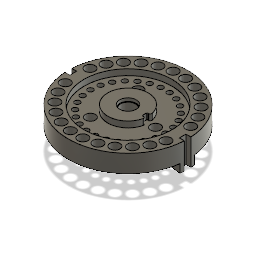
Reverse Roll v5 (Autodesk Fusion 360 design; units mm, degrees)
Autodesk Fusion 360 part; units mm, degrees
sketch "View A" plane through (0, 0, 0) normal (0, 1, 0) x (1, 0, 0)
  circle A0 centre (0, 0) radius 26.45
  circle A1 centre (0, 0) radius 16.6 construction
  circle A2 centre (0, 0) radius 22.6 construction
  circle A3 centre (0, 0) radius 31.25 construction
  circle A4 centre (16.6, 0) radius 3
  circle A5 centre (-8.3, 14.376) radius 3
  circle A6 centre (-8.3, -14.376) radius 3
  circle A7 centre (0, 0) radius 5
  circle A8 centre (0, 0) radius 4.5
  line L0 (10.5, 1.5) -> (10.9174, 1.5)
  line L1 (10.9174, -1.5) -> (10.5, -1.5)
  line L2 (10, -1) -> (10, 1)
  arc A9 (10.5, 1.5) -> (10, 1) centre (10.5, 1) ccw
  arc A10 (10, -1) -> (10.5, -1.5) centre (10.5, -1) ccw
  arc A11 (10.9174, 1.5) -> (11.8922, 2.7232) centre (10.9174, 2.5) ccw
  arc A12 (11.8922, -2.7232) -> (10.9174, -1.5) centre (10.9174, -2.5) ccw
  circle A13 centre (-22.5979, 0) radius 1.6
  circle A14 centre (-22.5979, 0) radius 2
  circle A15 centre (-21.9412, -5.408) radius 2
  circle A16 centre (-21.9412, -5.408) radius 1.6
  circle A17 centre (-20.0094, -10.5017) radius 2
  circle A18 centre (-20.0094, -10.5017) radius 1.6
  circle A19 centre (-16.9148, -14.9851) radius 2
  circle A20 centre (-16.9148, -14.9851) radius 1.6
  circle A21 centre (-12.8371, -18.5977) radius 2
  circle A22 centre (-12.8371, -18.5977) radius 1.6
  circle A23 centre (-8.0133, -21.1294) radius 2
  circle A24 centre (-8.0133, -21.1294) radius 1.6
  circle A25 centre (-2.7239, -22.4331) radius 2
  circle A26 centre (-2.7239, -22.4331) radius 1.6
  circle A27 centre (2.7239, -22.4331) radius 2
  circle A28 centre (2.7239, -22.4331) radius 1.6
  circle A29 centre (8.0133, -21.1294) radius 2
  circle A30 centre (8.0133, -21.1294) radius 1.6
  circle A31 centre (12.837, -18.5977) radius 2
  circle A32 centre (12.837, -18.5977) radius 1.6
  circle A33 centre (16.9147, -14.9852) radius 2
  circle A34 centre (16.9147, -14.9852) radius 1.6
  circle A35 centre (20.0094, -10.5018) radius 2
  circle A36 centre (20.0094, -10.5018) radius 1.6
  circle A37 centre (21.9412, -5.408) radius 2
  circle A38 centre (21.9412, -5.408) radius 1.6
  circle A39 centre (22.5979, 0) radius 2
  circle A40 centre (22.5979, 0) radius 1.6
  circle A41 centre (21.9412, 5.408) radius 2
  circle A42 centre (21.9412, 5.408) radius 1.6
  circle A43 centre (20.0094, 10.5017) radius 2
  circle A44 centre (20.0094, 10.5017) radius 1.6
  circle A45 centre (16.9148, 14.9851) radius 2
  circle A46 centre (16.9148, 14.9851) radius 1.6
  circle A47 centre (12.8371, 18.5977) radius 2
  circle A48 centre (12.8371, 18.5977) radius 1.6
  circle A49 centre (8.0133, 21.1294) radius 2
  circle A50 centre (8.0133, 21.1294) radius 1.6
  circle A51 centre (2.7239, 22.4331) radius 2
  circle A52 centre (2.7239, 22.4331) radius 1.6
  circle A53 centre (-2.7239, 22.4331) radius 2
  circle A54 centre (-2.7239, 22.4331) radius 1.6
  circle A55 centre (-8.0133, 21.1294) radius 2
  circle A56 centre (-8.0133, 21.1294) radius 1.6
  circle A57 centre (-12.837, 18.5977) radius 2
  circle A58 centre (-12.837, 18.5977) radius 1.6
  circle A59 centre (-16.9147, 14.9852) radius 2
  circle A60 centre (-16.9147, 14.9852) radius 1.6
  circle A61 centre (-20.0094, 10.5018) radius 2
  circle A62 centre (-20.0094, 10.5018) radius 1.6
  circle A63 centre (-21.9412, 5.408) radius 2
  circle A64 centre (-21.9412, 5.408) radius 1.6
  circle A65 centre (-31.25, -0.0368) radius 3 construction
  circle A66 centre (-30.3331, -7.5143) radius 3
  circle A67 centre (-27.6534, -14.5552) radius 3
  circle A68 centre (-23.3665, -20.7501) radius 3
  circle A69 centre (-17.7217, -25.7391) radius 3
  circle A70 centre (-11.047, -29.2323) radius 3
  circle A71 centre (-3.7302, -31.0266) radius 3
  circle A72 centre (3.8033, -31.0177) radius 3
  circle A73 centre (11.1158, -29.2062) radius 3
  circle A74 centre (17.7823, -25.6973) radius 3
  circle A75 centre (23.4153, -20.695) radius 3
  circle A76 centre (27.6876, -14.49) radius 3
  circle A77 centre (30.3507, -7.4429) radius 3
  circle A78 centre (31.25, 0.0368) radius 3 construction
  circle A79 centre (30.3331, 7.5143) radius 3
  circle A80 centre (27.6534, 14.5552) radius 3
  circle A81 centre (23.3665, 20.7501) radius 3
  circle A82 centre (17.7217, 25.7391) radius 3
  circle A83 centre (11.047, 29.2323) radius 3
  circle A84 centre (3.7302, 31.0266) radius 3
  circle A85 centre (-3.8033, 31.0177) radius 3
  circle A86 centre (-11.1158, 29.2062) radius 3
  circle A87 centre (-17.7823, 25.6973) radius 3
  circle A88 centre (-23.4153, 20.695) radius 3
  circle A89 centre (-27.6876, 14.49) radius 3
  circle A90 centre (-30.3507, 7.4429) radius 3
  line L3 (-35.9464, 1.9631) -> (-32.9464, 1.9631)
  line L4 (-32.9464, 1.9631) -> (-32.9464, -2.0369)
  line L5 (-32.9464, -2.0369) -> (-35.9423, -2.0369)
  line L6 (35.9464, -1.9631) -> (32.9464, -1.9631)
  line L7 (32.9464, -1.9631) -> (32.9464, 2.0369)
  line L8 (32.9464, 2.0369) -> (35.9423, 2.0369)
  arc A91 (-35.9423, -2.0369) -> (35.9464, -1.9631) centre (0, 0) ccw
  arc A92 (35.9423, 2.0369) -> (-35.9464, 1.9631) centre (0, 0) ccw
  circle A93 centre (0, 0) radius 8.5 construction
  arc A94 (0, 8.5) -> (-4.25, 7.3612) centre (0, 0) ccw
  line L9 (0, 0) -> (0, 8.5) construction
  line L10 (0, 0) -> (-4.25, 7.3612) construction
  circle A95 centre (-4.25, 7.3612) radius 3
  circle A96 centre (-4.25, -7.3612) radius 3
  circle A97 centre (8.5, 0) radius 3
  circle A98 centre (0, 0) radius 12.2
  dimension "d1" = 24.4
  dimension "d2" = 52.9
  dimension "d7" = 6
  dimension "d9" = 360
  dimension "d16" = 0.5
  dimension "d18" = 1
  dimension "d19" = 1
  dimension "d21" = 0.5
  dimension "d25" = 360
  dimension "d26" = 6
  dimension "d28" = 360
  dimension "d30" = 4
  dimension "d32" = 4
  dimension "d37" = 17
  dimension "d38" = 30
  dimension "d39" = 6
  dimension "d41" = 360
  dimension "d126" = 3
  dimension "d127" = 3
  measures "d1" diameter of A98
  measures "d2" diameter of A0
  measures "d7" diameter of A4
  measures "d16" radius of A9
  measures "d18" radius of A11
  measures "d19" radius of A12
  measures "d21" radius of A10
  measures "d26" diameter of A65
  measures "d37" diameter of A93
  measures "d38" angle of L9 L10
  measures "d39" diameter of A95
sketch "View B" plane through (0, 0, 0) normal (0, 1, 0) x (1, 0, 0)
  circle A0 centre (0, 0) radius 12.5
  circle A1 centre (0, 0) radius 17 construction
  circle A2 centre (-15.9748, 5.8143) radius 2
  circle A3 centre (13.0228, 10.9274) radius 2
  circle A4 centre (2.952, -16.7417) radius 2
  arc A5 (-35.9423, -2.0369) -> (35.9464, -1.9631) centre (0, 0) ccw
  line L0 (35.7317, -4.3873) -> (26.7445, -3.2838)
  line L1 (26.175, -3.8044) -> (20.7581, -3.0171)
  line L2 (24.9681, -8.729) -> (19.801, -6.9225)
  line L3 (26.7445, 3.2838) -> (35.7317, 4.3873)
  line L4 (25.3133, -2.4374) -> (14.8977, -1.4345)
  line L5 (25.3133, 2.4374) -> (14.8977, 1.4345)
  arc A6 (26.4075, -1.4987) -> (26.4075, 1.4987) centre (0, 0) ccw
  arc A7 (26.4075, 1.4987) -> (25.3133, 2.4374) centre (25.4091, 1.442) ccw
  arc A8 (25.3133, -2.4374) -> (26.4075, -1.4987) centre (25.4091, -1.442) ccw
  arc A9 (20.7581, -3.0171) -> (19.6326, -3.8159) centre (20.6142, -4.0067) ccw
  arc A10 (19.1724, -5.6938) -> (19.6326, -3.8159) centre (0, 0) ccw
  arc A11 (19.1724, -5.6938) -> (19.801, -6.9225) centre (20.131, -5.9785) ccw
  arc A12 (26.7445, -3.2838) -> (26.1885, -3.71) centre (26.6836, -3.7801) ccw
  arc A13 (26.1885, 3.71) -> (26.7445, 3.2838) centre (26.6836, 3.7801) ccw
  line L6 (-25.3133, -2.4374) -> (-14.8977, -1.4345)
  line L7 (-25.3133, 2.4374) -> (-14.8977, 1.4345)
  arc A14 (-25.3133, 2.4374) -> (-26.4075, 1.4987) centre (-25.4091, 1.442) ccw
  arc A15 (-26.4075, 1.4987) -> (-26.4075, -1.4987) centre (0, 0) ccw
  arc A16 (-26.4075, -1.4987) -> (-25.3133, -2.4374) centre (-25.4091, -1.442) ccw
  line L8 (-35.7317, 4.3873) -> (-26.7445, 3.2838)
  line L9 (-26.7445, -3.2838) -> (-35.7317, -4.3873)
  arc A17 (-26.1885, -3.71) -> (-26.7445, -3.2838) centre (-26.6836, -3.7801) ccw
  arc A18 (-26.7445, 3.2838) -> (-26.1885, 3.71) centre (-26.6836, 3.7801) ccw
  arc A19 (-26.1885, -3.71) -> (26.1885, -3.71) centre (0, 0) ccw
  arc A20 (26.1885, 3.71) -> (-26.1885, 3.71) centre (0, 0) ccw
  arc A21 (-26.4075, 1.4987) -> (-26.4075, -1.4987) centre (0, 0) ccw
  line L10 (26.1647, 3.8742) -> (20.7499, 3.0724)
  arc A22 (19.6224, 3.8682) -> (20.7499, 3.0724) centre (20.6035, 4.0616) ccw
  arc A23 (19.6224, 3.8682) -> (19.1571, 5.7449) centre (0, 0) ccw
  arc A24 (19.7825, 6.9752) -> (19.1571, 5.7449) centre (20.115, 6.0321) ccw
  line L11 (24.9448, 8.7955) -> (19.7825, 6.9752)
  line L12 (24.4773, 10.0232) -> (19.4117, 7.9489)
  arc A25 (18.1264, 8.4517) -> (19.4117, 7.9489) centre (19.0328, 8.8743) ccw
  arc A26 (18.1264, 8.4517) -> (17.2256, 10.1626) centre (0, 0) ccw
  arc A27 (17.5383, 11.5068) -> (17.2256, 10.1626) centre (18.0869, 10.6707) ccw
  line L13 (22.115, 14.5096) -> (17.5383, 11.5068)
  line L14 (21.3673, 15.5898) -> (16.9453, 12.3635)
  arc A28 (15.5771, 12.5441) -> (16.9453, 12.3635) centre (16.3559, 13.1713) ccw
  arc A29 (15.5771, 12.5441) -> (14.293, 13.9896) centre (0, 0) ccw
  arc A30 (14.275, 15.3696) -> (14.293, 13.9896) centre (15.0077, 14.6891) ccw
  line L15 (18.0001, 19.3804) -> (14.275, 15.3696)
  line L16 (17.0155, 20.2503) -> (13.4942, 16.0595)
  arc A31 (12.1224, 15.9074) -> (13.4942, 16.0595) centre (12.7286, 16.7028) ccw
  arc A32 (12.1224, 15.9074) -> (10.5298, 17.0037) centre (0, 0) ccw
  arc A33 (10.182, 18.3392) -> (10.5298, 17.0037) centre (11.0562, 17.8538) ccw
  line L17 (12.839, 23.1249) -> (10.182, 18.3392)
  line L18 (11.6749, 23.7339) -> (9.2588, 18.8222)
  arc A34 (7.9633, 18.3463) -> (9.2588, 18.8222) centre (8.3615, 19.2636) ccw
  arc A35 (7.9633, 18.3463) -> (6.1545, 19.0295) centre (0, 0) ccw
  arc A36 (5.4972, 20.243) -> (6.1545, 19.0295) centre (6.4623, 19.981) ccw
  line L19 (6.9317, 25.5255) -> (5.4972, 20.243)
  line L20 (5.6557, 25.8382) -> (4.4853, 20.491)
  arc A37 (3.3413, 19.7189) -> (4.4853, 20.491) centre (3.5084, 20.7049) ccw
  arc A38 (3.3413, 19.7189) -> (1.4216, 19.9494) centre (0, 0) ccw
  arc A39 (0.493, 20.9704) -> (1.4216, 19.9494) centre (1.4927, 20.9469) ccw
  line L21 (0.6217, 26.4427) -> (0.493, 20.9704)
  line L22 (-0.6921, 26.4409) -> (-0.5489, 20.969)
  arc A40 (-1.4748, 19.9456) -> (-0.5489, 20.969) centre (-1.5485, 20.9428) ccw
  arc A41 (-1.4748, 19.9456) -> (-3.3939, 19.7099) centre (0, 0) ccw
  arc A42 (-4.5399, 20.479) -> (-3.3939, 19.7099) centre (-3.5636, 20.6954) ccw
  line L23 (-5.7246, 25.8231) -> (-4.5399, 20.479)
  line L24 (-6.9997, 25.507) -> (-5.5511, 20.2283)
  arc A43 (-6.2052, 19.013) -> (-5.5511, 20.2283) centre (-6.5155, 19.9637) ccw
  arc A44 (-6.2052, 19.013) -> (-8.0121, 18.325) centre (0, 0) ccw
  arc A45 (-9.3089, 18.7975) -> (-8.0121, 18.325) centre (-8.4128, 19.2412) ccw
  line L25 (-11.7381, 23.7027) -> (-9.3089, 18.7975)
  line L26 (-12.9006, 23.0907) -> (-10.2308, 18.312)
  arc A46 (-10.575, 16.9755) -> (-10.2308, 18.312) centre (-11.1038, 17.8243) ccw
  arc A47 (-10.575, 16.9755) -> (-12.1648, 15.8751) centre (0, 0) ccw
  arc A48 (-13.5369, 16.0235) -> (-12.1648, 15.8751) centre (-12.773, 16.6688) ccw
  line L27 (-17.0694, 20.2049) -> (-13.5369, 16.0235)
  line L28 (-18.0516, 19.3324) -> (-14.3159, 15.3315)
  arc A49 (-14.3302, 13.9515) -> (-14.3159, 15.3315) centre (-15.0468, 14.6491) ccw
  arc A50 (-14.3302, 13.9515) -> (-15.6105, 12.5025) centre (0, 0) ccw
  arc A51 (-16.9782, 12.3183) -> (-15.6105, 12.5025) centre (-16.391, 13.1277) ccw
  line L29 (-21.4088, 15.5328) -> (-16.9782, 12.3183)
  line L30 (-22.1536, 14.4506) -> (-17.5689, 11.46)
  arc A52 (-17.2526, 10.1166) -> (-17.5689, 11.46) centre (-18.1153, 10.6225) ccw
  arc A53 (-17.2526, 10.1166) -> (-18.1489, 8.4034) centre (0, 0) ccw
  arc A54 (-19.4328, 7.8972) -> (-18.1489, 8.4034) centre (-19.0563, 8.8236) ccw
  line L31 (-24.5039, 9.958) -> (-19.4328, 7.8972)
  line L32 (-24.9681, 8.729) -> (-19.801, 6.9225)
  arc A55 (-19.1724, 5.6938) -> (-19.801, 6.9225) centre (-20.131, 5.9785) ccw
  arc A56 (-19.1724, 5.6938) -> (-19.6326, 3.8159) centre (0, 0) ccw
  arc A57 (-20.7581, 3.0171) -> (-19.6326, 3.8159) centre (-20.6142, 4.0067) ccw
  line L33 (-26.175, 3.8044) -> (-20.7581, 3.0171)
  line L34 (-26.1647, -3.8742) -> (-20.7499, -3.0724)
  arc A58 (-19.6224, -3.8682) -> (-20.7499, -3.0724) centre (-20.6035, -4.0616) ccw
  arc A59 (-19.6224, -3.8682) -> (-19.1571, -5.7449) centre (0, 0) ccw
  arc A60 (-19.7825, -6.9752) -> (-19.1571, -5.7449) centre (-20.115, -6.0321) ccw
  line L35 (-24.9448, -8.7955) -> (-19.7825, -6.9752)
  line L36 (-24.4773, -10.0232) -> (-19.4117, -7.9489)
  arc A61 (-18.1264, -8.4517) -> (-19.4117, -7.9489) centre (-19.0328, -8.8743) ccw
  arc A62 (-18.1264, -8.4517) -> (-17.2256, -10.1626) centre (0, 0) ccw
  arc A63 (-17.5383, -11.5068) -> (-17.2256, -10.1626) centre (-18.0869, -10.6707) ccw
  line L37 (-22.115, -14.5096) -> (-17.5383, -11.5068)
  line L38 (-21.3673, -15.5898) -> (-16.9453, -12.3635)
  arc A64 (-15.5771, -12.5441) -> (-16.9453, -12.3635) centre (-16.3559, -13.1713) ccw
  arc A65 (-15.5771, -12.5441) -> (-14.293, -13.9896) centre (0, 0) ccw
  arc A66 (-14.275, -15.3696) -> (-14.293, -13.9896) centre (-15.0077, -14.6891) ccw
  line L39 (-18.0001, -19.3804) -> (-14.275, -15.3696)
  line L40 (-17.0155, -20.2503) -> (-13.4942, -16.0595)
  arc A67 (-12.1224, -15.9074) -> (-13.4942, -16.0595) centre (-12.7286, -16.7028) ccw
  arc A68 (-12.1224, -15.9074) -> (-10.5298, -17.0037) centre (0, 0) ccw
  arc A69 (-10.182, -18.3392) -> (-10.5298, -17.0037) centre (-11.0562, -17.8538) ccw
  line L41 (-12.839, -23.1249) -> (-10.182, -18.3392)
  line L42 (-11.6749, -23.7339) -> (-9.2588, -18.8222)
  arc A70 (-7.9633, -18.3463) -> (-9.2588, -18.8222) centre (-8.3615, -19.2636) ccw
  arc A71 (-7.9633, -18.3463) -> (-6.1545, -19.0295) centre (0, 0) ccw
  arc A72 (-5.4972, -20.243) -> (-6.1545, -19.0295) centre (-6.4623, -19.981) ccw
  line L43 (-6.9317, -25.5255) -> (-5.4972, -20.243)
  line L44 (-5.6557, -25.8382) -> (-4.4853, -20.491)
  arc A73 (-3.3413, -19.7189) -> (-4.4853, -20.491) centre (-3.5084, -20.7049) ccw
  arc A74 (-3.3413, -19.7189) -> (-1.4216, -19.9494) centre (0, 0) ccw
  arc A75 (-0.493, -20.9704) -> (-1.4216, -19.9494) centre (-1.4927, -20.9469) ccw
  line L45 (-0.6217, -26.4427) -> (-0.493, -20.9704)
  line L46 (0.6921, -26.4409) -> (0.5489, -20.969)
  arc A76 (1.4748, -19.9456) -> (0.5489, -20.969) centre (1.5485, -20.9428) ccw
  arc A77 (1.4748, -19.9456) -> (3.3939, -19.7099) centre (0, 0) ccw
  arc A78 (4.5399, -20.479) -> (3.3939, -19.7099) centre (3.5636, -20.6954) ccw
  line L47 (5.7246, -25.8231) -> (4.5399, -20.479)
  line L48 (6.9997, -25.507) -> (5.5511, -20.2283)
  arc A79 (6.2052, -19.013) -> (5.5511, -20.2283) centre (6.5155, -19.9637) ccw
  arc A80 (6.2052, -19.013) -> (8.0121, -18.325) centre (0, 0) ccw
  arc A81 (9.3089, -18.7975) -> (8.0121, -18.325) centre (8.4128, -19.2412) ccw
  line L49 (11.7381, -23.7027) -> (9.3089, -18.7975)
  line L50 (12.9006, -23.0907) -> (10.2308, -18.312)
  arc A82 (10.575, -16.9755) -> (10.2308, -18.312) centre (11.1038, -17.8243) ccw
  arc A83 (10.575, -16.9755) -> (12.1648, -15.8751) centre (0, 0) ccw
  arc A84 (13.5369, -16.0235) -> (12.1648, -15.8751) centre (12.773, -16.6688) ccw
  line L51 (17.0694, -20.2049) -> (13.5369, -16.0235)
  line L52 (18.0516, -19.3324) -> (14.3159, -15.3315)
  arc A85 (14.3302, -13.9515) -> (14.3159, -15.3315) centre (15.0468, -14.6491) ccw
  arc A86 (14.3302, -13.9515) -> (15.6105, -12.5025) centre (0, 0) ccw
  arc A87 (16.9782, -12.3183) -> (15.6105, -12.5025) centre (16.391, -13.1277) ccw
  line L53 (21.4088, -15.5328) -> (16.9782, -12.3183)
  line L54 (22.1536, -14.4506) -> (17.5689, -11.46)
  arc A88 (17.2526, -10.1166) -> (17.5689, -11.46) centre (18.1153, -10.6225) ccw
  arc A89 (17.2526, -10.1166) -> (18.1489, -8.4034) centre (0, 0) ccw
  arc A90 (19.4328, -7.8972) -> (18.1489, -8.4034) centre (19.0563, -8.8236) ccw
  line L55 (24.5039, -9.958) -> (19.4328, -7.8972)
  arc A91 (13.8151, 2.2679) -> (-13.8151, 2.2679) centre (0, 0) ccw
  arc A92 (-13.8151, -2.2679) -> (13.8151, -2.2679) centre (0, 0) ccw
  arc A93 (-14.8977, 1.4345) -> (-13.8151, 2.2679) centre (-14.8019, 2.4299) ccw
  arc A94 (-13.8151, -2.2679) -> (-14.8977, -1.4345) centre (-14.8019, -2.4299) ccw
  arc A95 (14.8977, -1.4345) -> (13.8151, -2.2679) centre (14.8019, -2.4299) ccw
  arc A96 (13.8151, 2.2679) -> (14.8977, 1.4345) centre (14.8019, 2.4299) ccw
  line L56 (-32.9464, 1.9631) -> (-32.9464, -2.0369)
  line L57 (-35.9464, 1.9631) -> (-32.9464, 1.9631)
  line L58 (-32.9464, -2.0369) -> (-35.9423, -2.0369)
  line L59 (32.9464, -1.9631) -> (32.9464, 2.0369)
  line L60 (35.9464, -1.9631) -> (32.9464, -1.9631)
  line L61 (32.9464, 2.0369) -> (35.9423, 2.0369)
  arc A97 (-35.9423, -2.0369) -> (35.9464, -1.9631) centre (0, 0) ccw
  arc A98 (35.9423, 2.0369) -> (-35.9464, 1.9631) centre (0, 0) ccw
  dimension "d54" = 25
  dimension "d56" = 34
  dimension "d63" = 4
  dimension "d64" = 4
  dimension "d65" = 4
  dimension "d71" = 1
  dimension "d72" = 1
  dimension "d73" = 1
  dimension "d74" = 1
  dimension "d75" = 0.5
  dimension "d76" = 0.5
  dimension "d80" = 360
  dimension "d81" = 1
  measures "d54" diameter of A0
  measures "d56" diameter of A1
  measures "d63" diameter of A2
  measures "d64" diameter of A3
  measures "d65" diameter of A4
  measures "d71" radius of A7
  measures "d72" radius of A8
  measures "d73" radius of A9
  measures "d74" radius of A11
  measures "d75" radius of A12
  measures "d76" radius of A13
  measures "d81" radius of A93
extrude "Extrude8" add sketch "View B" along normal blind 20.9 contours A0
extrude "Extrude9" cut sketch "View A" along normal blind 6 contours L0 L1 L2 A9 A10 A11 A12 A97 | L0 L1 L2 A9 A10 A11 A12 A97 | A95 | A96
extrude "Extrude10" add sketch "View A" along normal blind 24.5 contours L0 L1 L2 A9 A10 A11 A12 A97 | A11 A12 A97 A98 | A95 | A96 picked at (8.5028, 0.0746) picked at (-7.5975, -3.0679)
extrude "Extrude11" cut sketch "View A" along normal blind 6 contours L0 L1 L2 A9 A10 A11 A12 A97 | L0 L1 L2 A9 A10 A11 A12 A97 | A95 | A96
extrude "Extrude12" cut sketch "View A" along normal blind 31 contours A8
extrude "Extrude13" add sketch "View A" along normal blind 6 from surface at 14.9 contours A0
extrude "Extrude14" add sketch "View A" along normal blind 3.4 from surface at 11.5 contours A0 | A4 | A5 | A6
extrude "Extrude15" add sketch "View A" along normal blind 9.4 from surface at 11.5 contours A14 | A15 | A17 | A19 | A21 | A23 | A25 | A27 | A29 | A31 | A33 | A35 | A37 | A39 | A41 | A43 | A45 | A47 | A49 | A51 | A53 | A55 | A57 | A59 | A61 | A63
extrude "Extrude16" add sketch "View A" against normal blind 10.8 from surface at 24.5 contours L3 L4 L5 L6 L7 L8 A91 A92
extrude "Extrude17" add sketch "View B" along normal blind 6 from surface at 8.5 contours A5 L0 L1 L2 L3 A9 A10 A11 A12 A13 L8 L9 A17 A18 A19 A20 L10 A22 A23 A24 L11 L12 A25 A26 A27 L13 L14 A28 A29 A30 L15 L16 A31 A32 A33 L17 L18 A34 A35 A36 L19 L20 A37 A38 A39 L21 L22 A40 A41 A42 L23 L24 A43 A44 A45 L25 L26 A46 A47 A48 L27 L28 A49 A50 A51 L29 L30 A52 A53 A54 L31 L32 A55 A56 A57 L33 L34 A58 A59 A60 L35 L36 A61 A62 A63 L37 L38 A64 A65 A66 L39 L40 A67 A68 A69 L41 L42 A70 A71 A72 L43 L44 A73 A74 A75 L45 L46 A76 A77 A78 L47 L48 A79 A80 A81 L49 L50 A82 A83 A84 L51 L52 A85 A86 A87 L53 L54 A88 A89 A90 L55 L56 L57 L58 L59 L60 L61 A97 A98
extrude "Extrude18" cut sketch "View B" along normal blind 3.5 from surface at 8.5 contours A2 | A3 | A4
extrude "Extrude19" cut sketch "View A" along normal blind 1 from surface at 11.5 contours A14 | A15 | A17 | A19 | A21 | A23 | A25 | A27 | A29 | A31 | A33 | A35 | A37 | A39 | A41 | A43 | A45 | A47 | A49 | A51 | A53 | A55 | A57 | A59 | A61 | A63
extrude "Extrude20" add sketch "View A" along normal blind 22.6 contours A7
extrude "Extrude21" add sketch "View B" against normal blind 1 from surface at 11.5 contours L4 L5 A6 A7 A8 L6 L7 A14 A15 A16 A21 A91 A92 A93 A94 A95 A96
extrude "Extrude22" cut sketch "View A" along normal blind 16 contours A13 | A16 | A18 | A20 | A22 | A24 | A26 | A28 | A30 | A32 | A34 | A36 | A38 | A40 | A42 | A44 | A46 | A48 | A50 | A52 | A54 | A56 | A58 | A60 | A62 | A64
extrude "Extrude23" add sketch "View A" along normal blind 3 from surface at 10.5 contours A14 | A39
extrude "Extrude24" cut sketch "View A" along normal blind 1 from surface at 10.5 contours A14 | A39
extrude "Extrude25" add sketch "View B" against normal blind 1 from surface at 11.5 contours A19 L34 A58 A59 A60 L35 | L1 L2 A9 A10 A11 A19 | A19 L36 A61 A62 A63 L37 | A19 L54 A88 A89 A90 L55 | A20 L32 A55 A56 A57 L33 | A19 L38 A64 A65 A66 L39 | A20 L10 A22 A23 A24 L11 | A19 L52 A85 A86 A87 L53 | A20 L30 A52 A53 A54 L31 | A19 L40 A67 A68 A69 L41 | A20 L12 A25 A26 A27 L13 | A19 L50 A82 A83 A84 L51 | A20 L28 A49 A50 A51 L29 | A19 L42 A70 A71 A72 L43 | A20 L14 A28 A29 A30 L15 | A19 L48 A79 A80 A81 L49 | A20 L26 A46 A47 A48 L27 | A19 L44 A73 A74 A75 L45 | A20 L16 A31 A32 A33 L17 | A19 L46 A76 A77 A78 L47 | A20 L24 A43 A44 A45 L25 | A20 L18 A34 A35 A36 L19 | A20 L22 A40 A41 A42 L23 | A20 L20 A37 A38 A39 L21
extrude "Extrude26" add sketch "View A" along normal blind 2 from surface at 10.5 contours A15 | A17 | A19 | A21 | A23 | A25 | A27 | A29 | A31 | A33 | A35 | A37 | A41 | A43 | A45 | A47 | A49 | A51 | A53 | A55 | A57 | A59 | A61 | A63
extrude "Extrude27" cut sketch "View A" along normal blind 1 from surface at 10.5 contours A15 | A17 | A19 | A21 | A23 | A25 | A27 | A29 | A31 | A33 | A35 | A37 | A41 | A43 | A45 | A47 | A49 | A51 | A53 | A55 | A57 | A59 | A61 | A63
extrude "Extrude28" cut sketch "View A" along normal blind 25 contours A16 | A18 | A20 | A22 | A24 | A26 | A28 | A30 | A32 | A34 | A36 | A38 | A42 | A44 | A46 | A48 | A50 | A52 | A54 | A56 | A58 | A60 | A62 | A64
equation "d37 = ( 8.5 * 2 ) * 1 mm"
equation "d82 = 24.5 mm - 3.6 mm"
equation "d92 = 24.5 mm - 9.6 mm"
equation "d93 = 9.6 mm - 3.6 mm"
equation "d95 = 24.5 mm - 16 mm + 2 mm + 1 mm"
equation "d96 = 16 mm - 9.6 mm - 2 mm - 1 mm"
equation "d98 = 24.5 mm - 16 mm + 2 mm + 1 mm"
equation "d104 = 24.5 mm - 16 mm"
equation "d113 = 24.5 mm - 1.9 mm"
equation "d116 = -3.00 mm + 2 mm"
